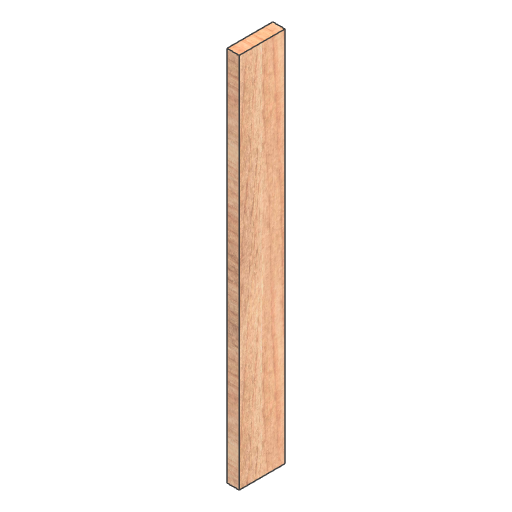
# Autodesk Inventor part: CUT PART P-01
Saved by Autodesk Inventor 2023.2 (Build 272271000, 271)
## iProperties
Created: 2022-11-14
Part Number: CUT PART P-01
Material: Wood (Birch)
Document SubType Name: Modeling
Designer: GUT
Density: 0.55 g/cm^3
Appearance: Birch - Natural Polished
Mass: 109.89 g
Surface Area: 432.6 cm^2
Volume: 199.8 cm^3
d0: 370,000 mm
Author: GUT
Autodesk Inventor part; units mm, degrees
ref_plane "YZ Plane" through (0, 0, 0) normal (1, 0, 0) x (0, 1, 0)
ref_plane "XZ Plane" through (0, 0, 0) normal (0, 1, 0) x (-1, 0, 0)
ref_plane "XY Plane" through (0, 0, 0) normal (0, 0, 1) x (1, 0, 0)
sketch "Sketch1" plane through (0, 0, 0) normal (1, 0, 0) x (0, 1, 0)
  line L0 (429.5129, 174.9923) -> (59.5129, 174.9923)
  line L1 (59.5129, 174.9923) -> (59.5129, 219.9923)
  line L2 (59.5129, 219.9923) -> (429.5129, 219.9923)
  line L3 (429.5129, 219.9923) -> (429.5129, 174.9923)
  point P0 (0, 0)
  dimension "d0" = 370
  dimension "d1" = 45
  constraints: 8 end point, 2 parallel, 1 horizontal, 1 perpendicular
  measures "d0" distance of L0.start L0.end
  measures "d1" distance of L0.end L1.end
extrude "Extrusion1" add sketch "Sketch1" along normal blind 12
body "Solid1"
